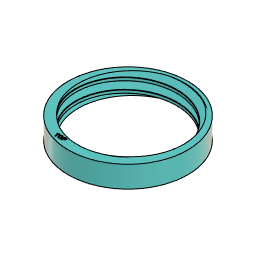
cap assembly v5 (Autodesk Fusion 360 archive; units mm, degrees)
design "battery cap"
Autodesk Fusion 360 part; units mm, degrees
note: some values were not read from the file. Chosen so that the rebuilt part matches the saved one: which face or edge a step refers to.
sketch "Sketch3" plane through (0, 0, 0) normal (0, 0, 1) x (1, 0, 0) in component "cap"
  circle A0 centre (0, 0) radius 21.75
  circle A1 centre (0, 0) radius 27.75
  dimension "d49" = 43.5
  dimension "d50" = 6
  constraint coincident A0.centre A1.centre
  measures "d49" diameter of A0
extrude "Extrude2" add sketch "Sketch3" along normal blind 10 makes body 1 in component "cap"
thread "Thread1" "ISO Metric profile 52.0 M52x5 6H" major diameter 52.5183 minor diameter 46.9423 pitch 5 angle 60 modelled right hand crest width 1.364 on face at (21.723, -1.0841, 6.6667) crest through (23.4712, 0, 1.25) on bodies 1 in component "cap"
fillet "Fillet1" radius 0.2 5 edges at (8.1998, -21.9922, 0.966) (0, 23.4712, 8.182) (-21.9922, -8.1998, 9.716) (0, 23.4712, 3.182) (0, -23.4712, 5.682) on bodies 1 in component "cap"
sketch "emboss" plane through (0, 0, 10) normal (0, 0, 1) x (-1, 0, 0)
  spline S0 degree 3 poles (18.8897, 14.099) (18.5438, 14.51) (18.0705, 15.0742) (16.7805, 16.4512) (16.079, 17.127) (15.3313, 17.772) knots 0 0 0 0 0.161158 0.161158 0.34023 0.34023 0.34023 0.34023
  spline S1 degree 3 poles (18.8897, 14.099) (20.5039, 12.1809) (21.804, 10.014) (23.9232, 4.7546) (24.5132, 1.6245) (24.4727, -4.7565) (23.8162, -7.9453) (21.3025, -13.962) (19.4454, -16.7214) (15.6843, -20.4844) (14.0883, -21.7412) (10.6148, -23.8706) (8.7463, -24.7306) (6.7967, -25.3643) knots 0.171284 0.171284 0.171284 0.171284 0.925537 0.925537 1.871553 1.871553 2.83804 2.83804 3.824988 3.824988 4.431164 4.431164 5.044877 5.044877 5.044877 5.044877
  arc A0 (-6.7967, -25.3643) -> (6.7967, -25.3643) centre (0, 0) ccw
  spline S2 degree 3 poles (-6.7967, -25.3643) (-10.012, -24.3192) (-12.9945, -22.6624) (-18.0957, -18.3334) (-20.1819, -15.7233) (-23.1933, -9.9057) (-24.1127, -6.7666) (-24.6775, -0.3803) (-24.3437, 2.8028) (-22.8453, 7.6258) (-22.0789, 9.3501) (-20.1686, 12.5601) (-19.0364, 14.0377) (-17.7419, 15.3662) knots 0 0 0 0 1.014256 1.014256 2.008013 2.008013 2.981262 2.981262 3.933998 3.933998 4.499168 4.499168 5.056789 5.056789 5.056789 5.056789
  arc A1 (15.3313, 17.772) -> (-17.7419, 15.3662) centre (0, 0) ccw
  circle A2 centre (0, 0) radius 27.75
  line L0 (9.4086, 26.2544) -> (0, 26.2544) construction
  line L1 (0, 26.2544) -> (0, 23.4093) construction
  line L2 (0, 23.4093) -> (9.4086, 23.4093) construction
  line L3 (9.4086, 23.4093) -> (9.4086, 26.2544) construction
  spline S3 degree 3 poles (-6.7967, -25.3643) (-1.8106, -26.7004) (3.5707, -26.5224) (8.4577, -24.8598) (13.3429, -23.1978) (17.7149, -20.0587) (20.8515, -15.9612) (23.987, -11.865) (25.8755, -6.8272) (26.2054, -1.6792) (26.5352, 3.4671) (25.306, 8.703) (22.7206, 13.165) (20.136, 17.6256) (16.2063, 21.295) (11.5793, 23.5683) (6.856, 25.8889) (1.425, 26.7434) (-3.7827, 25.9853) (-8.912, 25.2386) (-13.8036, 22.9318) (-17.6428, 19.4493) (-21.478, 15.9703) (-24.2475, 11.3319) (-25.4909, 6.3053) (-26.7331, 1.2835) (-26.4471, -4.1057) (-24.6804, -8.9678) (-22.9152, -13.8257) (-19.679, -18.1382) (-15.508, -21.1907) (-11.3404, -24.2407) (-6.256, -26.0207) (-1.096, -26.2363) (4.0602, -26.4517) (9.2714, -25.1041) (13.6769, -22.4162) (18.0794, -19.7301) (21.6598, -15.7161) (23.8273, -11.0364) (26.0734, -6.1872) (26.7897, -0.6429) (25.8499, 4.6179) (24.9391, 9.7163) (22.4793, 14.5275) (18.8796, 18.2511) (15.2866, 21.9679) (10.5723, 24.5864) (5.5182, 25.6728) (0.472, 26.7574) (-4.8929, 26.3105) (-9.69, 24.4059) (-14.481, 22.5037) (-18.6868, 19.1551) (-21.6141, 14.9122) (-24.5511, 10.6553) (-26.1892, 5.5149) (-26.2569, 0.3436) (-26.3244, -4.8122) (-24.8307, -9.9783) (-22.0223, -14.3025) (-19.2121, -18.6296) (-15.0965, -22.0966) (-10.3551, -24.1312) (-9.2005, -24.6267) (-8.0103, -25.0391) (-6.7967, -25.3643) knots 13.87535334 13.87535334 13.87535334 13.87535334 14.46509837 14.46509837 14.46509837 15.05463416 15.05463416 15.05463416 15.64397098 15.64397098 15.64397098 16.23311907 16.23311907 16.23311907 16.82208862 16.82208862 16.82208862 17.42331583 17.42331583 17.42331583 18.01549272 18.01549272 18.01549272 18.60706737 18.60706737 18.60706737 19.1980824 19.1980824 19.1980824 19.78858002 19.78858002 19.78858002 20.37860205 20.37860205 20.37860205 20.96818995 20.96818995 20.96818995 21.5573849 21.5573849 21.5573849 22.16792728 22.16792728 22.16792728 22.75962192 22.75962192 22.75962192 23.35022171 23.35022171 23.35022171 23.93989451 23.93989451 23.93989451 24.52880539 24.52880539 24.52880539 25.11965578 25.11965578 25.11965578 25.70873565 25.70873565 25.70873565 26.29818622 26.29818622 26.29818622 26.44172395 26.44172395 26.44172395 26.44172395
  dimension "d55" = 1.7
  text T0 "TOP" font "Arial" height 1.7 bold align left top in box 9.4086 x 2.8451 at (9.4086, 26.2544) x (-1, 0) y (0, -1) spacing 1 kerned
  constraint coincident S3
emboss "Emboss1" depth -2 profiles "emboss" section 1 text T0 onto face at (11.4266, -23.6568, 10) on bodies 1 bodies 1 makes body 2 at (-5.6885, -24.0185, 8.9852) in component "cap"
sketch "Sketch4" plane through (0, 0, 0) normal (0, 0, -1) x (1, 0, 0)
  spline S0 degree 3 poles (-15.3313, 17.772) (-16.0788, 17.1272) (-16.7802, 16.4515) (-18.0702, 15.0745) (-18.5437, 14.5101) (-18.8897, 14.099) knots 0 0 0 0 0.296149 0.296149 0.562854 0.562854 0.562854 0.562854
  arc A0 (17.7419, 15.3662) -> (-15.3313, 17.772) centre (0, 0) ccw
  spline S1 degree 3 poles (17.7419, 15.3662) (19.8949, 13.1566) (21.5905, 10.5438) (23.9232, 4.7546) (24.5132, 1.6245) (24.4727, -4.7565) (23.8162, -7.9453) (21.3025, -13.962) (19.4454, -16.7214) (15.6843, -20.4844) (14.0883, -21.7412) (10.6148, -23.8706) (8.7463, -24.7306) (6.7967, -25.3643) knots 0 0 0 0 0.925537 0.925537 1.871553 1.871553 2.83804 2.83804 3.824988 3.824988 4.431164 4.431164 5.044877 5.044877 5.044877 5.044877
  arc A1 (-6.7967, -25.3643) -> (6.7967, -25.3643) centre (0, 0) ccw
  spline S2 degree 3 poles (-6.7967, -25.3643) (-10.012, -24.3192) (-12.9945, -22.6624) (-18.0957, -18.3334) (-20.1819, -15.7233) (-23.1933, -9.9057) (-24.1127, -6.7666) (-24.6775, -0.3803) (-24.3437, 2.8028) (-22.8453, 7.6258) (-22.0789, 9.3501) (-20.4604, 12.0698) (-19.7155, 13.1177) (-18.8897, 14.099) knots 0 0 0 0 1.014256 1.014256 2.008013 2.008013 2.981262 2.981262 3.933998 3.933998 4.499168 4.499168 4.88528 4.88528 4.88528 4.88528
  circle A2 centre (0, 0) radius 27.75
  line L0 (-3.2029, 23.9916) -> (4.3966, 23.9916) construction
  line L1 (4.3966, 23.9916) -> (4.3966, 26.2544) construction
  line L2 (4.3966, 26.2544) -> (-3.2029, 26.2544) construction
  line L3 (-3.2029, 26.2544) -> (-3.2029, 23.9916) construction
  dimension "d60" = 1.7
  text T0 "BOTTOM\n" font "Arial" height 1.7 bold align left top in box 7.5995 x 2.2628 at (-3.2029, 23.9916) x (1, 0) y (0, 1) spacing 1 kerned
emboss "Emboss2" depth -2 profiles "Sketch4" section 1 text T0 onto face at (11.4266, -23.6568, 0) on bodies 1 bodies 1 makes body 3 at (-2.8596, -25.1439, 1.0717) in component "cap"
component "cap" placed x (1, 0, 0) y (0, 1, 0) z (0, 0, 1) at (0, 0, 0)
equation "LDO_length = 44 mm"
equation "LDO_width = 21 mm"
equation "LDO_depth = 12 mm"
equation "battery_length = 60 mm"
equation "battery_width = 39 mm"
equation "battery_depth = 10 mm"
equation "shell = 1.5 mm"
equation "gap = 0.2 mm"
equation "fillet = 2 mm"
equation "thread_height = 10 mm"
equation "thread_offset_fix = 0.2 mm"
equation "battery_holder_id = battery_width + 3 * shell"
equation "thread_od = battery_holder_id + 3 * shell"
equation "scd30_width = 51 mm"
equation "scd30_length = 25.4 mm"
equation "scd30_depth = 8.8 mm"
equation "wemos_mini_width = 31 mm"
equation "wemos_mini_length = 39 mm"
equation "wemos_mini_depth = 4.15 mm"
equation "d49 = battery_holder_id"
equation "d50 = shell * 4"
equation "d51 = thread_height"
equation "d54 = thread_offset_fix"
equation "d55 = shell + gap"
equation "d60 = shell + gap"
named bodies: "battery cap", "TOP emboss", "BOTTOM emboss"
